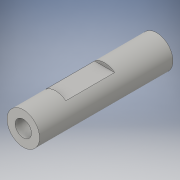
# Autodesk Inventor part: Pin V2
Saved by Autodesk Inventor 2016 (Build 200138000, 138)
## iProperties
Created: 2015-08-06
Part Number: Pin V2
Material: Generic
Document SubType Name: Modeling
Designer: Jason
Density: 1 g/cm^3
Appearance: Default
Author: Jason
Autodesk Inventor part; units mm, degrees
ref_plane "XZ Plane" through (0, 0, 0) normal (0, 1, 0) x (-1, 0, 0)
ref_plane "XY Plane" through (0, 0, 0) normal (0, 0, 1) x (1, 0, 0)
sketch "Sketch1" plane through (0, 0, 0) normal (0, 0, 1) x (1, 0, 0)
  circle A0 centre (0, 0) radius 6.35
  dimension "d0" = 12.7
  constraints: 1 centre point, 1 coincident
  measures "d0" diameter of A0
extrude "Extrusion1" add sketch "Sketch1" along normal blind 52.07
ref_plane "Work Plane1" through (-6.35, 0, 0) normal (1, 0, 0) x (0, 1, 0)
sketch "Sketch2" plane through (-6.35, 0, 0) normal (1, 0, 0) x (0, 1, 0)
  line L0 (-6.35, 0) -> (6.35, 0) projected
  line L1 (6.35, 52.07) -> (-6.35, 52.07) projected
  line L2 (6.35, 0) -> (6.35, 52.07) projected
  line L3 (-6.35, 0) -> (-6.35, 52.07) projected
  line L4 (6.35, 20.32) -> (5, 20.32)
  line L5 (5, 20.32) -> (5, 39.37)
  line L6 (5, 39.37) -> (6.35, 39.37)
  line L7 (6.35, 39.37) -> (6.35, 20.32)
  line L8 (-6.35, 20.32) -> (-5, 20.32)
  line L9 (-5, 20.32) -> (-5, 39.37)
  line L10 (-5, 39.37) -> (-6.35, 39.37)
  line L11 (-6.35, 39.37) -> (-6.35, 20.32)
  point P0 (0, 0)
  dimension "d3" = 19.05
  dimension "d4" = 12.7
  dimension "d5" = 10
  constraints: 16 end point, 4 parallel, 2 collinear, 2 horizontal, 2 perpendicular, 2 point on line
  measures "d3" distance of L4.end L5.end
  measures "d4" distance between parallel lines of L1 L6
  measures "d5" distance between parallel lines of L9 L5
extrude "Extrusion2" cut sketch "Sketch2" along normal mid plane 52.07 contours L3 L10 L9 L8 | L4 L5 L6 L2
sketch "Sketch3" plane through (0, 0, 52.07) normal (0, 0, 1) x (1, 0, 0)
  point P0 (0, 0)
  point P1 (0, 0)
  constraints: 1 coincident
hole "Hole1" at (0, 0, 52.07) direction (0, 0, -1) diameter 6.35 depth 25.4 tip angle 118
body "Solid1"
